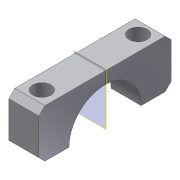
# Autodesk Inventor part: Halterung_Motor
Saved by Autodesk Inventor 2015 (Build 190159000, 159)
## iProperties
Created: 2015-08-08
Part Number: Halterung_Motor
Material: ABS-Kunststoff
Document SubType Name: Modeling
Designer: Johann
Density: 1.06 g/cm^3
Appearance: Glatt - weiß
Mass: 0.502609 g
Surface Area: 6.79957 cm^2
Volume: 0.474159 cm^3
Author: Johann
Autodesk Inventor part; units mm, degrees
ref_plane "YZ Plane" through (0, 0, 0) normal (1, 0, 0) x (0, 1, 0)
ref_plane "XY Plane" through (0, 0, 0) normal (0, 0, 1) x (1, 0, 0)
sketch "Skizze1" plane through (0, 0, 0) normal (1, 0, 0) x (0, 1, 0)
  line L0 (-11, 0) -> (-6, 0)
  arc A0 (6, 0) -> (-6, 0) centre (0, 0) ccw
  line L1 (6, 0) -> (11, 0)
  line L2 (11, 0) -> (11, 8)
  line L3 (-11, 8) -> (-11, 0)
  line L4 (-11, 8) -> (11, 8)
  point P0 (0, 0)
  dimension "d2" = 6
  dimension "d18" = 22
  dimension "d26" = 8
  constraints: 10 end point, 3 point on line, 2 horizontal, 2 point on circle, 1 centre point, 1 coincident, 1 collinear, 1 perpendicular, 1 vertical
  measures "d2" radius of A0
  measures "d18" distance between parallel lines of L2 L3
  measures "d26" distance from line of L4 point (0, 0)
extrude "Extrusion1" add sketch "Skizze1" along normal mid plane 5
ref_plane "Arbeitsebene2" through (0, 0, 0) normal (1, 0, 0) x (0, 0, -1)
sketch "Skizze5" plane through (2.5, -6, 0) normal (0, 0, -1) x (-1, 0, 0)
  line L0 (2.5, 6) -> (-2.4006, 6) construction
  line L1 (0, -5) -> (0, 0) projected
  point P0 (2.5, -2)
  point P1 (2.5, 14)
  dimension "d27" = 16
  dimension "d28" = 2.5
  constraints: 2 end point, 1 horizontal, 1 symmetric about line
  measures "d27" distance of point (2.5, 14) point (2.5, -2)
  measures "d28" distance from line of point (2.5, -2) L1
hole "Bohrung2" at (0, -8, 0) at (0, 8, 0) direction (0, 0, 1) diameter 3 end through all
chamfer "Fase1" distance 1 angle 45 4 edges at (0, -11, 8) (0, 11, 8) (0, 11, 0) (0, -11, 0)
